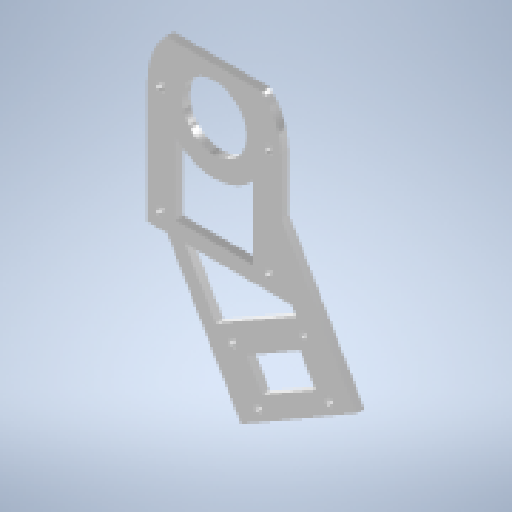
# Autodesk Inventor part: elbow
Saved by Autodesk Inventor 2024.1 (Build 281209000, 209)
## iProperties
Created: 2024-02-14
Part Number: elbow
Material: アルミニウム 6061
Document SubType Name: Modeling
Designer: hibik
Density: 2.7 g/cm^3
Appearance: アルミニウム - フラット
Author: hibik
Autodesk Inventor part; units mm, degrees
ref_plane "YZ Plane" through (0, 0, 0) normal (1, 0, 0) x (0, 1, 0)
ref_plane "XZ Plane" through (0, 0, 0) normal (0, 1, 0) x (-1, 0, 0)
ref_plane "XY Plane" through (0, 0, 0) normal (0, 0, 1) x (1, 0, 0)
sketch "スケッチ2" plane through (0, 0, 0) normal (0, 0, 1) x (1, 0, 0)
  line L0 (0, 0) -> (26, 0)
  line L1 (26, 0) -> (26, 33)
  line L2 (26, 33) -> (0, 33)
  line L3 (0, 33) -> (0, 0)
  line L4 (0, 0) -> (26, 0)
  line L5 (26, 0) -> (26, 24)
  line L6 (26, 24) -> (0, 24) construction
  line L7 (0, 24) -> (0, 0)
  circle A0 centre (13, 24) radius 13
  circle A1 centre (13, 24) radius 6.25
  line L8 (26, 0) -> (0, 0)
  line L9 (17.9352, 27.452) -> (40.6962, -11.9711)
  line L10 (40.6962, -11.9711) -> (18.1795, -24.9711)
  line L11 (18.1795, -24.9711) -> (-4.3205, 14)
  circle A2 centre (21.5096, -20.7391) radius 0.8
  circle A3 centre (35.366, -12.7391) radius 0.8
  line L12 (-4.3205, 14) -> (18.1962, 27)
  point P0 (22.3808, 33)
  point P1 (3.6192, 33)
  point P2 (26, 13.4833)
  point P3 (3.7624, 0)
  point P4 (23.9624, 17.0125)
  point P5 (1.7417, 17.5)
  point P6 (0, 16.4944)
  point P7 (0, 6.5167)
  point P8 (7.5873, 20.875)
  point P9 (19.0712, 25.4845)
  dimension "d0" = 26
  dimension "d1" = 33
  dimension "d2" = 24
  dimension "d3" = 12.5
  dimension "d14" = 26
  dimension "d17" = 1.6
  dimension "d18" = 1.6
  dimension "d19" = 2
  dimension "d20" = 2
  dimension "d21" = 5
  dimension "d22" = 5
  dimension "d23" = 20
  dimension "d25" = 45
  dimension "d26" = 30
  constraints: 26 end point, 5 parallel, 3 centre point, 3 horizontal, 3 perpendicular, 3 point on line, 1 coincident, 1 midpoint, 3 other
  measures "d0" distance of L1.end L2.end
  measures "d1" distance of L2.end L0.start
  measures "d2" distance between parallel lines of L0 L6
  measures "d3" diameter of A1
  measures "d14" distance between parallel lines of L11 L9
  measures "d17" diameter of A2
  measures "d18" diameter of A3
  measures "d19" distance from line of A2.centre L10
  measures "d20" distance from line of L10 A3.centre
  measures "d21" distance from line of L11 A2.centre
  measures "d22" distance from line of L9 A3.centre
  measures "d23" distance from line of L11 A1.centre
  measures "d25" distance between parallel lines of L10 L12
  measures "d26" angle of L9 L1
extrude "押し出し1" add sketch "スケッチ2" along normal blind 1.5 contours L3 L11 L0 | L11 L3 L12 A0 L9 L1 L0 | L0 L1 L9 L10 L11 | L3 A0 L12 | L9 A0 L1 | A0 L2 L9 A1 L12 | L12 A1 L9 A0
sketch "スケッチ3" plane through (0, 0, 0) normal (0, 0, -1) x (-1, 0, 0)
  circle A0 centre (-2.5, 24) radius 0.85 projected
  circle A1 centre (-23.5, 24) radius 0.85 projected
  circle A2 centre (-23.5, 3) radius 0.85 projected
  circle A3 centre (-2.5, 3) radius 0.85 projected
  circle A4 centre (-30.366, -4.0788) radius 0.8 projected
  circle A5 centre (-16.5096, -12.0788) radius 0.8 projected
  circle A6 centre (-13, 24) radius 6.25 projected
  line L0 (-2.5, 24) -> (-23.5, 24)
  line L1 (-23.5, 24) -> (-23.5, 3)
  line L2 (-23.5, 3) -> (-2.5, 3)
  line L3 (-2.5, 3) -> (-2.5, 24)
  circle A7 centre (-13, 24) radius 10.25
  line L4 (-5.5, 24) -> (-20.5, 24)
  line L5 (-20.5, 24) -> (-20.5, 3)
  line L6 (-20.5, 3) -> (-5.5, 3)
  line L7 (-5.5, 3) -> (-5.5, 24)
  line L8 (-3.7624, 0) -> (-18.1795, -24.9711) projected
  line L9 (0, 24) -> (0, 0) projected
  arc A8 (0, 24) -> (-3.6192, 33) centre (-13, 24) ccw projected
  line L10 (-22.3808, 33) -> (-3.6192, 33) projected
  arc A9 (-22.3808, 33) -> (-26, 24) centre (-13, 24) ccw projected
  line L11 (-26, 13.4833) -> (-26, 24) projected
  line L12 (-40.6962, -11.9711) -> (-26, 13.4833) projected
  line L13 (-18.1795, -24.9711) -> (-40.6962, -11.9711) projected
  line L14 (-3.7624, 0) -> (-18.1795, -24.9711) projected
  line L15 (0, 0) -> (-3.7624, 0) projected
  circle A10 centre (-13, 24) radius 6.25 projected
  circle A11 centre (-21.5096, -20.7391) radius 0.8 projected
  circle A12 centre (-35.366, -12.7391) radius 0.8 projected
  line L16 (-21.5096, -20.7391) -> (-16.5096, -12.0788)
  line L17 (-16.5096, -12.0788) -> (-30.366, -4.0788)
  line L18 (-30.366, -4.0788) -> (-35.366, -12.7391)
  line L19 (-35.366, -12.7391) -> (-21.5096, -20.7391)
  line L20 (-22.2417, -18.007) -> (-19.2417, -12.8109)
  line L21 (-19.2417, -12.8109) -> (-29.634, -6.8109)
  line L22 (-29.634, -6.8109) -> (-32.634, -12.007)
  line L23 (-32.634, -12.007) -> (-22.2417, -18.007)
  line L24 (-13.2817, -10.4784) -> (-24.5317, -3.9832)
  line L25 (-24.5317, -3.9832) -> (-16.75, 9.4952)
  line L26 (-16.75, 9.4952) -> (-5.5, 3)
  line L27 (-5.5, 3) -> (-13.2817, -10.4784)
  line L28 (-24.5317, -3.9832) -> (-28.866, -1.4808)
  line L29 (-28.866, -1.4808) -> (-28.0111, 0)
  line L30 (-28.0111, 0) -> (-22.2321, 0)
  line L31 (-22.2321, 0) -> (-7.2321, 0)
  point P0 (-5.5, 17.0134)
  point P1 (-20.5, 17.0134)
  dimension "d27" = 4
  dimension "d28" = 3
  dimension "d29" = 3
  dimension "d31" = 2
  dimension "d32" = 2
  dimension "d33" = 2
  dimension "d34" = 2
  dimension "d35" = 3
  dimension "d36" = 3
  constraints: 48 end point, 12 parallel, 6 perpendicular, 5 point on line, 4 coincident, 3 horizontal, 2 collinear, 1 centre point
  measures "d27" radial gap between concentric circles of A7 A6
  measures "d28" distance between parallel lines of L3 L7
  measures "d29" distance between parallel lines of L1 L5
  measures "d31" distance between parallel lines of L19 L23
  measures "d32" distance between parallel lines of L17 L21
  measures "d33" distance between parallel lines of L16 L20
  measures "d34" distance between parallel lines of L18 L22
  measures "d35" distance between parallel lines of L17 L24
  measures "d36" distance from line of L1.end L30
extrude "押し出し2" cut sketch "スケッチ3" against normal through all contours A0 L3 L0 A7 | A7 L0 A0 | A0 A7 L0 L3 | L0 A7 A0 | L3 L2 A3 | A3 L2 L3 | L7 L26 L25 L5 A7 | A7 L0 L1 A1 | A1 L0 A7 | L2 L25 L26 | A1 A7 L0 | L1 L0 A7 A1 | L27 L24 L25 L31 | L1 L2 A2 | A2 L2 L1 | L25 L28 L29 L30 | A4 L17 L18 | L18 L17 A4 | L17 L16 A5 | A5 L16 L17 | L23 L22 L21 L20
fillet "フィレット1" radius 3 19 edges at (20.5, 3, 0.75) (5.5, 3, 0.75) (20.5, 17.0134, 0.75) (5.5, 17.0134, 0.75) (7.2321, 0, 0.75) (13.2817, -10.4784, 0.75) (28.0111, 0, 0.75) (28.866, -1.4808, 0.75) (29.634, -6.8109, 0.75) (32.634, -12.007, 0.75) (22.2417, -18.007, 0.75) (19.2417, -12.8109, 0.75) (40.6962, -11.9711, 0.75) (18.1795, -24.9711, 0.75) (3.7624, 0, 0.75) (0, 0, 0.75) (26, 13.4833, 0.75) (22.3808, 33, 0.75) (3.6192, 33, 0.75)
equation "\"d20\" = d19"
